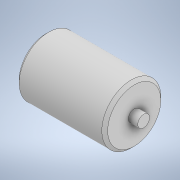
# Autodesk Inventor part: 零件4
Saved by Autodesk Inventor 2020 (Build 240168000, 168)
## iProperties
Created: 2020-12-28
Part Number: 零件4
Material: 一般
Document SubType Name: Modeling
Designer: User
Density: 1 g/cm^3
Appearance: 預設
Author: User
Autodesk Inventor part; units mm, degrees
ref_plane "YZ Plane" through (0, 0, 0) normal (1, 0, 0) x (0, 1, 0)
ref_plane "XZ Plane" through (0, 0, 0) normal (0, 1, 0) x (-1, 0, 0)
ref_plane "XY Plane" through (0, 0, 0) normal (0, 0, 1) x (1, 0, 0)
sketch "草圖1" plane through (0, 0, 0) normal (0, 0, 1) x (1, 0, 0)
  line L0 (0, 0) -> (0, 1143)
  line L1 (127, 1270) -> (3683, 1270)
  line L2 (3810, 1143) -> (3810, 0)
  line L3 (3810, 0) -> (0, 0)
  line L4 (3810, 0) -> (3810, 254)
  line L5 (3810, 254) -> (4216.4, 254)
  line L6 (4216.4, 254) -> (4216.4, 0)
  line L7 (4216.4, 0) -> (3810, 0)
  line L8 (0, 0) -> (0, 254)
  line L9 (0, 254) -> (-406.4, 254)
  line L10 (-406.4, 254) -> (-406.4, 0)
  line L11 (-406.4, 0) -> (0, 0)
  line L12 (3.175, 1270) -> (0, 1266.825)
  line L13 (127, 1270) -> (0, 1143)
  line L14 (3683, 1270) -> (3810, 1143)
  point P0 (0, 1270)
  point P1 (3810, 1270)
  point P2 (0, 1270)
  dimension "d0" = 1270
  dimension "d1" = 3810
  dimension "d2" = 254
  dimension "d3" = 406.4
  dimension "d4" = 406.4
  dimension "d5" = 3.175
  dimension "d6" = 3.175
  dimension "d7" = 127
  dimension "d8" = 127
  dimension "d9" = 127
  dimension "d10" = 127
  constraints: 30 end point, 14 point on line, 8 perpendicular, 1 vertical
  measures "d0" distance of L0.start point (0, 1270)
  measures "d1" distance of point (0, 1270) point (3810, 1270)
  measures "d2" distance of L2.end L4.end
  measures "d3" distance of L4.end L5.end
  measures "d4" distance of L8.end L9.end
  measures "d5" distance of L12.start point (0, 1270)
  measures "d6" distance of L12.end point (0, 1270)
  measures "d7" distance of L1.start point (0, 1270)
  measures "d8" distance of L0.end point (0, 1270)
  measures "d9" distance of L1.end point (3810, 1270)
  measures "d10" distance of L2.start point (3810, 1270)
revolve "迴轉1" add sketch "草圖1" angle 360 about axis through (3810, 0, 0) along (-1, 0, 0)
equation "\"d6\" = d5"
equation "\"d8\" = d7"
equation "\"d9\" = d7"
equation "\"d10\" = d9"
